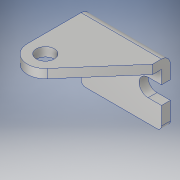
# Autodesk Inventor part: LeftAngleBracket-1111-2018
Saved by Autodesk Inventor 2017 (Build 210142000, 142)
## iProperties
Created: 2018-02-10
Part Number: LeftAngleBracket-1111-2018
Material: Aluminum 6061
Document SubType Name: Modeling
Designer: Phyllis
Density: 2.7 g/cm^3
Appearance: Aluminum - Flat
Author: Phyllis
Autodesk Inventor part; units mm, degrees
ref_plane "YZ Plane" through (0, 0, 0) normal (1, 0, 0) x (0, 1, 0)
ref_plane "XZ Plane" through (0, 0, 0) normal (0, 1, 0) x (-1, 0, 0)
ref_plane "XY Plane" through (0, 0, 0) normal (0, 0, 1) x (1, 0, 0)
sketch "Sketch1" plane through (0, 0, 0) normal (0, 0, 1) x (1, 0, 0)
  line L0 (0, 0) -> (28.575, 0)
  line L1 (28.575, 0) -> (28.575, 19.05)
  line L2 (28.575, 19.05) -> (0, 19.05)
  line L3 (0, 19.05) -> (0, 0)
  arc A0 (23.8125, 14.2875) -> (23.8125, 7.9375) centre (23.8125, 11.1125) ccw
  arc A1 (4.7625, 7.9375) -> (4.7625, 14.2875) centre (4.7625, 11.1125) ccw
  line L4 (0, 7.9375) -> (4.7625, 7.9375)
  line L5 (0, 14.2875) -> (4.7625, 14.2875)
  line L6 (28.575, 14.2875) -> (23.8125, 14.2875)
  line L7 (28.575, 7.9375) -> (23.8125, 7.9375)
  dimension "d4" = 28.575
  dimension "d5" = 19.05
  dimension "d18" = 7.9375
  dimension "d19" = 4.7625
  dimension "d20" = 7.9375
  dimension "d21" = 4.7625
  dimension "d22" = 6.35
  dimension "d23" = 6.35
  dimension "d24" = 4.7625
  dimension "d25" = 4.7625
  dimension "d26" = 4.7625
  dimension "d27" = 4.7625
  constraints: 16 end point, 4 point on circle, 4 point on line, 4 tangent, 2 centre point, 2 parallel, 1 horizontal, 1 perpendicular
  measures "d4" distance of L0.start L0.end
  measures "d5" distance of L0.end L1.end
  measures "d18" distance from line of L2 A0.centre
  measures "d19" distance from line of A0.centre L1
  measures "d20" distance from line of L2 A1.centre
  measures "d21" horizontal distance of L2.end A1.centre
  measures "d22" diameter of A1
  measures "d23" diameter of A0
  measures "d24" horizontal distance of L5.end L2.end
  measures "d25" distance of L4.start L4.end
  measures "d26" distance of L6.start L6.end
  measures "d27" distance of L7.start L7.end
extrude "Extrusion1" add sketch "Sketch1" along normal blind 3.175
sketch "Sketch3" plane through (0, 19.05, 0) normal (0, 1, 0) x (1, 0, 0)
  line L0 (0, 0) -> (28.575, 0) projected
  line L1 (0, 0) -> (28.575, 0)
  line L2 (28.575, 0) -> (28.575, -6.35)
  line L3 (28.575, -6.35) -> (0, -6.35)
  line L4 (0, 0) -> (0, -3.175) projected
  line L5 (0, 0) -> (0, -22.225)
  circle A0 centre (6.35, -22.225) radius 6.35
  line L6 (28.575, -6.35) -> (11.1411, -26.3925)
  circle A1 centre (6.35, -22.225) radius 3.175
  dimension "d6" = 6.35
  dimension "d8" = 22.225
  dimension "d10" = 28.575
  dimension "d12" = 12.7
  dimension "d13" = 6.35
  dimension "d16" = 6.35
  constraints: 10 end point, 2 centre point, 2 coincident, 2 point on circle, 1 horizontal, 1 parallel, 1 perpendicular, 1 tangent, 1 vertical
  measures "d6" distance between parallel lines of L0 L3
  measures "d8" distance from line of L0 point (6.35, -22.225)
  measures "d10" distance from line of L2 L0.start
  measures "d12" diameter of A0
  measures "d13" horizontal distance of point (6.35, -22.225) L0.start
  measures "d16" diameter of A1
extrude "Extrusion2" add sketch "Sketch3" along normal blind 3.175
fillet "Fillet1" radius 3.175 1 edges at (14.2875, 22.225, 0)
sketch "Sketch4" plane through (0, 0, 0) normal (0, 0, -1) x (-1, 0, 0)
  arc A0 (-23.8125, 7.9375) -> (-23.8125, 14.2875) centre (-23.8125, 11.1125) ccw
  arc A1 (-4.7625, 14.2875) -> (-4.7625, 7.9375) centre (-4.7625, 11.1125) ccw
  line L0 (-28.575, 19.05) -> (0, 19.05) projected
  line L1 (-28.575, 0) -> (-28.575, 19.05) projected
  line L2 (0, 0) -> (0, 19.05) projected
  line L3 (-28.575, 0) -> (-28.575, 19.05) projected
  line L4 (-28.575, 14.2875) -> (-23.8125, 14.2875)
  line L5 (-28.575, 7.9375) -> (-23.8125, 7.9375)
  line L6 (0, 19.05) -> (0, 0) projected
  line L7 (0, 14.2875) -> (-4.7625, 14.2875)
  line L8 (0, 7.9375) -> (-4.7625, 7.9375)
  dimension "d28" = 6.35
  dimension "d29" = 6.35
  dimension "d30" = 7.9375
  dimension "d31" = 7.9375
  dimension "d32" = 4.7625
  dimension "d33" = 4.7625
  dimension "d34" = 4.7625
  dimension "d35" = 4.7625
  dimension "d36" = 4.7625
  dimension "d38" = 4.7625
  constraints: 8 end point, 4 point on circle, 4 point on line, 4 tangent, 2 centre point
  measures "d28" diameter of A0
  measures "d29" diameter of A1
  measures "d30" distance from line of L0 A0.centre
  measures "d31" distance from line of L0 A1.centre
  measures "d32" distance from line of A0.centre L1
  measures "d33" distance from line of A1.centre L2
  measures "d34" distance of L4.start L4.end
  measures "d35" distance of L5.start L5.end
  measures "d36" distance of L7.start L7.end
  measures "d38" distance of L8.start L8.end
extrude "Extrusion3" cut sketch "Sketch4" against normal through all
fillet "Fillet2" radius 1.5875 2 edges at (28.575, 0, 1.5875) (0, 0, 1.5875)
equation "\"d23\" = d22"
equation "\"d24\" = d21"
equation "\"d26\" = d19"
equation "\"d27\" = d19"
equation "\"d29\" = d28"
equation "\"d31\" = d30"
equation "\"d34\" = d32"
equation "\"d35\" = d32"
equation "\"d36\" = d33"
equation "\"d38\" = d33"
body "Solid1"
